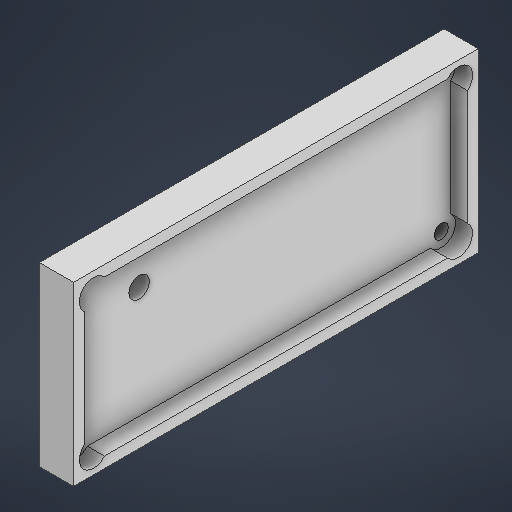
# Autodesk Inventor part: wb_box2026_lid1
Saved by Autodesk Inventor 2027.1 (Build 311270010, 270A)
## iProperties
Created: 2022-08-26
Part Number: wb_box2026_lid1
Material: Générique
Document SubType Name: Modeling
Designer: PCA
Density: 1 g/cm^3
Appearance: Par défaut
Author: PCA
Autodesk Inventor part; units mm, degrees
ref_plane "YZ Plane" through (0, 0, 0) normal (1, 0, 0) x (0, 1, 0)
ref_plane "XZ Plane" through (0, 0, 0) normal (0, 1, 0) x (-1, 0, 0)
ref_plane "XY Plane" through (0, 0, 0) normal (0, 0, 1) x (1, 0, 0)
sketch "Esquisse1" plane through (0, 0, 0) normal (1, 0, 0) x (0, 1, 0)
  line L0 (-15.5, -35.5) -> (15.5, -35.5)
  line L1 (15.5, -35.5) -> (15.5, 35.5)
  line L2 (15.5, 35.5) -> (-15.5, 35.5)
  line L3 (-15.5, 35.5) -> (-15.5, -35.5)
  line L4 (-15.5, -35.5) -> (15.5, 35.5) construction
  line L5 (15.5, -35.5) -> (-15.5, 35.5) construction
  point P0 (0, 0)
  dimension "d0" = 31
  dimension "d1" = 71
  constraints: 12 end point, 2 midpoint, 2 parallel, 1 horizontal, 1 perpendicular
  measures "d0" distance of L2.end L1.end
  measures "d1" distance of L1.end L0.end
extrude "Extrusion1" add sketch "Esquisse1" against normal blind 6
sketch "Esquisse2" plane through (0, 0, 0) normal (1, 0, 0) x (0, 0, -1)
  line L0 (33.6, -13.6) -> (-33.6, -13.6)
  line L1 (-33.6, -13.6) -> (-33.6, 13.6)
  line L2 (-33.6, 13.6) -> (33.6, 13.6)
  line L3 (33.6, 13.6) -> (33.6, -13.6)
  line L4 (33.6, -13.6) -> (-33.6, 13.6) construction
  line L5 (-33.6, -13.6) -> (33.6, 13.6) construction
  point P0 (0, 0)
  dimension "d4" = 67.2
  dimension "d5" = 27.2
  constraints: 12 end point, 2 midpoint, 2 parallel, 1 horizontal, 1 perpendicular
  measures "d4" distance of L1.end L2.end
  measures "d5" distance of L0.end L1.end
extrude "Extrusion2" cut sketch "Esquisse2" against normal blind 3
sketch "Esquisse3" plane through (0, 0, 0) normal (1, 0, 0) x (0, 0, -1)
  line L0 (32, -12) -> (-32, 12) construction
  line L1 (-32, -12) -> (32, 12) construction
  arc A0 (-30.0791, 13.6) -> (-33.6, 10.0791) centre (-32, 12) ccw
  arc A1 (33.5, 10) -> (30, 13.5) centre (32, 12) ccw
  arc A2 (30.0791, -13.6) -> (33.6, -10.0791) centre (32, -12) ccw
  line L2 (-33.6, 13.6) -> (33.6, 13.6) projected
  line L3 (33.6, -13.6) -> (-33.6, 13.6) construction
  line L4 (-33.5, -13.5) -> (33.5, 13.5) construction
  arc A3 (-33.5, -10) -> (-30, -13.5) centre (-32, -12) ccw
  line L5 (-33.6, 13.6) -> (-30.0791, 13.6)
  line L6 (30, 13.5) -> (33.5, 13.5)
  line L7 (-33.5, -13.5) -> (-33.5, -10)
  line L8 (-33.6, 10.0791) -> (-33.6, 13.6)
  line L9 (33.6, -13.6) -> (30.0791, -13.6)
  line L10 (-30, -13.5) -> (-33.5, -13.5)
  line L11 (33.5, 13.5) -> (33.5, 10)
  line L12 (33.6, -10.0791) -> (33.6, -13.6)
  point P0 (0, 0)
  point P1 (33.5, 13.5)
  point P2 (30.0791, 13.6)
  point P3 (-30.0791, 13.6)
  dimension "d8" = 64
  dimension "d9" = 24
  dimension "d10" = 5
  dimension "d12" = 5
  dimension "d13" = 5
  constraints: 24 end point, 8 parallel, 8 point on circle, 4 centre point, 4 coincident, 4 midpoint, 4 perpendicular, 2 horizontal
  measures "d8" distance of L0.end L1.end
  measures "d9" distance of L1.start L0.end
  measures "d10" diameter of A0
  measures "d12" diameter of A1
  measures "d13" diameter of A2
extrude "Extrusion3" cut sketch "Esquisse3" against normal blind 3
sketch "Esquisse4" plane through (-6, 0, 0) normal (-1, 0, 0) x (0, 0, 1)
  line L0 (-28.9525, 9.2685) -> (3.8656, 9.2685) construction
  line L1 (3.8656, 9.2685) -> (3.8656, -1.9036) construction
  line L2 (3.8656, -1.9036) -> (-28.9525, -1.9036) construction
  line L3 (-28.9525, -1.9036) -> (-28.9525, 9.2685) construction
  line L4 (8.1238, -3.2547) -> (23.4156, -3.2547) construction
  line L5 (23.4156, -3.2547) -> (23.4156, -10.1675) construction
  line L6 (23.4156, -10.1675) -> (8.1238, -10.1675) construction
  line L7 (8.1238, -10.1675) -> (8.1238, -3.2547) construction
  line L8 (-28.297, 3.0616) -> (-28.297, 9.1616)
  line L9 (-28.297, 9.1616) -> (-25.9955, 9.1616)
  spline S0 degree 2 poles (-25.9955, 9.1616) (-25.3865, 9.1616) (-25.0657, 9.1012) knots 0 0 0 1 1 1
  spline S1 degree 2 poles (-25.0657, 9.1012) (-24.6147, 9.0268) (-24.0102, 8.6083) (-23.6383, 7.8505) (-23.6383, 7.3948) knots 0 0 0 1 2 3 3 3
  spline S2 degree 2 poles (-23.6383, 7.3948) (-23.6383, 6.6184) (-24.6286, 5.5397) (-25.9211, 5.5397) knots 0 0 0 1 2 2 2
  line L10 (-25.9211, 5.5397) -> (-27.488, 5.5397)
  line L11 (-27.488, 5.5397) -> (-27.488, 3.0616)
  line L12 (-27.488, 3.0616) -> (-28.297, 3.0616)
  line L13 (-27.488, 6.2604) -> (-25.9118, 6.2604)
  spline S3 degree 2 poles (-25.9118, 6.2604) (-25.1261, 6.2604) (-24.4705, 6.8416) (-24.4705, 7.3716) knots 0 0 0 1 2 2 2
  spline S4 degree 2 poles (-24.4705, 7.3716) (-24.4705, 7.7528) (-24.8564, 8.3015) (-25.1726, 8.3852) knots 0 0 0 1 2 2 2
  spline S5 degree 2 poles (-25.1726, 8.3852) (-25.3772, 8.441) (-25.9258, 8.441) knots 0 0 0 1 1 1
  line L14 (-25.9258, 8.441) -> (-27.488, 8.441)
  line L15 (-27.488, 8.441) -> (-27.488, 6.2604)
  line L16 (-18.2589, 5.205) -> (-17.45, 5.0004)
  spline S6 degree 2 poles (-17.45, 5.0004) (-17.7057, 4.0054) (-19.0214, 2.9593) (-19.9746, 2.9593) knots 0 0 0 1 2 2 2
  spline S7 degree 2 poles (-19.9746, 2.9593) (-20.9602, 2.9593) (-22.197, 3.7637) (-22.8432, 5.284) (-22.8432, 6.1581) knots 0 0 0 1 2 3 3 3
  spline S8 degree 2 poles (-22.8432, 6.1581) (-22.8432, 7.1112) (-22.1133, 8.5339) (-20.7696, 9.2685) (-19.9606, 9.2685) knots 0 0 0 1 2 3 3 3
  spline S9 degree 2 poles (-19.9606, 9.2685) (-19.0447, 9.2685) (-17.7987, 8.334) (-17.5522, 7.4925) knots 0 0 0 1 2 2 2
  line L17 (-17.5522, 7.4925) -> (-18.3473, 7.3019)
  spline S10 degree 2 poles (-18.3473, 7.3019) (-18.5612, 7.9667) (-19.3655, 8.5758) (-19.9792, 8.5758) knots 0 0 0 1 2 2 2
  spline S11 degree 2 poles (-19.9792, 8.5758) (-20.6813, 8.5758) (-21.6298, 7.9016) (-22.011, 6.7672) (-22.011, 6.1628) knots 0 0 0 1 2 3 3 3
  spline S12 degree 2 poles (-22.011, 6.1628) (-22.011, 5.3863) (-21.5554, 4.224) (-20.6022, 3.6521) (-20.0443, 3.6521) knots 0 0 0 1 2 3 3 3
  spline S13 degree 2 poles (-20.0443, 3.6521) (-19.3655, 3.6521) (-18.4263, 4.4332) (-18.2589, 5.205) knots 0 0 0 1 2 2 2
  line L18 (-17.1198, 3.0616) -> (-14.7766, 9.1616)
  line L19 (-14.7766, 9.1616) -> (-13.9025, 9.1616)
  line L20 (-13.9025, 9.1616) -> (-11.4104, 3.0616)
  line L21 (-11.4104, 3.0616) -> (-12.331, 3.0616)
  line L22 (-12.331, 3.0616) -> (-13.0377, 4.9074)
  line L23 (-13.0377, 4.9074) -> (-15.5948, 4.9074)
  line L24 (-15.5948, 4.9074) -> (-16.2644, 3.0616)
  line L25 (-16.2644, 3.0616) -> (-17.1198, 3.0616)
  line L26 (-15.3624, 5.563) -> (-13.2888, 5.563)
  line L27 (-13.2888, 5.563) -> (-13.9304, 7.2554)
  spline S14 degree 2 poles (-13.9304, 7.2554) (-14.2186, 8.0272) (-14.3581, 8.52) knots 0 0 0 1 1 1
  spline S15 degree 2 poles (-14.3581, 8.52) (-14.479, 7.9342) (-14.6882, 7.353) knots 0 0 0 1 1 1
  line L28 (-14.6882, 7.353) -> (-15.3624, 5.563)
  line L29 (8.0842, -9.3547) -> (10.1406, -3.2547)
  line L30 (10.1406, -3.2547) -> (11.1392, -3.2547)
  line L31 (11.1392, -3.2547) -> (13.1956, -9.3547)
  line L32 (13.1956, -9.3547) -> (12.3404, -9.3547)
  line L33 (12.3404, -9.3547) -> (11.7867, -7.6493)
  line L34 (11.7867, -7.6493) -> (9.4585, -7.6493)
  line L35 (9.4585, -7.6493) -> (8.9048, -9.3547)
  line L36 (8.9048, -9.3547) -> (8.0842, -9.3547)
  line L37 (11.5643, -6.9573) -> (10.6201, -4.0852)
  line L38 (10.6201, -4.0852) -> (9.6809, -6.9573)
  line L39 (9.6809, -6.9573) -> (11.5643, -6.9573)
  line L40 (18.2229, -9.3547) -> (17.17, -9.3547)
  line L41 (17.17, -9.3547) -> (14.9406, -6.5173)
  line L42 (14.9406, -6.5173) -> (14.5846, -6.9177)
  line L43 (14.5846, -6.9177) -> (14.5846, -9.3547)
  line L44 (14.5846, -9.3547) -> (13.7739, -9.3547)
  line L45 (13.7739, -9.3547) -> (13.7739, -3.2547)
  line L46 (13.7739, -3.2547) -> (14.5846, -3.2547)
  line L47 (14.5846, -3.2547) -> (14.5846, -6.0576)
  line L48 (14.5846, -6.0576) -> (17.0859, -3.2547)
  line L49 (17.0859, -3.2547) -> (18.0746, -3.2547)
  line L50 (18.0746, -3.2547) -> (15.5486, -5.9785)
  line L51 (15.5486, -5.9785) -> (18.2229, -9.3547)
  line L52 (18.0499, -9.3547) -> (20.1063, -3.2547)
  line L53 (20.1063, -3.2547) -> (21.1048, -3.2547)
  line L54 (21.1048, -3.2547) -> (23.1612, -9.3547)
  line L55 (23.1612, -9.3547) -> (22.306, -9.3547)
  line L56 (22.306, -9.3547) -> (21.7524, -7.6493)
  line L57 (21.7524, -7.6493) -> (19.4241, -7.6493)
  line L58 (19.4241, -7.6493) -> (18.8705, -9.3547)
  line L59 (18.8705, -9.3547) -> (18.0499, -9.3547)
  line L60 (21.5299, -6.9573) -> (20.5858, -4.0852)
  line L61 (20.5858, -4.0852) -> (19.6466, -6.9573)
  line L62 (19.6466, -6.9573) -> (21.5299, -6.9573)
  point P0 (0, 0)
  constraints: 4 other
extrude "Extrusion4" add sketch "Esquisse4" along normal blind 1
sketch "Esquisse5" plane through (-6, 0, 0) normal (-1, 0, 0) x (0, 0, 1)
  arc A0 (-30.0791, 13.6) -> (-33.6, 10.0791) centre (-32, 12) ccw projected
  line L0 (32, -12) -> (-32, -12)
  line L1 (-32, -12) -> (-32, 12)
  line L2 (-32, 12) -> (32, 12)
  line L3 (32, 12) -> (32, -12)
  line L4 (32, -12) -> (-32, 12) construction
  line L5 (-32, -12) -> (32, 12) construction
  circle A1 centre (-32, 12) radius 1.25
  circle A2 centre (-32, -12) radius 1.25
  circle A3 centre (32, 12) radius 1.25
  circle A4 centre (32, -12) radius 1.25
  line L6 (35.5, 15.5) -> (-35.5, 15.5) projected
  line L7 (35.5, -15.5) -> (35.5, 15.5) projected
  point P0 (0, 0)
  dimension "d18" = 64
  dimension "d19" = 24
  dimension "d20" = 2.5
  dimension "d21" = 2.5
  dimension "d22" = 2.5
  dimension "d24" = 2.5
  constraints: 12 end point, 4 centre point, 3 coincident, 2 midpoint, 2 parallel, 1 horizontal, 1 perpendicular, 1 point on line
  measures "d18" distance of L1.end L2.end
  measures "d19" distance of L0.end L1.end
  measures "d20" diameter of A1
  measures "d21" diameter of A2
  measures "d22" diameter of A3
  measures "d24" diameter of A4
hole "Perçage1" at (-6, 12, 32) at (-6, -12, -32) at (-6, -12, 32) at (-6, 12, -32) direction (1, 0, 0) diameter 2.5 end through all
sketch "Esquisse6" plane through (-6, 0, 0) normal (-1, 0, 0) x (0, 0, 1)
  circle A0 centre (21, 6) radius 1.8
  line L0 (35.5, 15.5) -> (-35.5, 15.5) projected
  line L1 (35.5, -15.5) -> (35.5, 15.5) projected
  point P0 (0, 0)
  dimension "d37" = 3.6
  dimension "d38" = 9.5
  dimension "d39" = 14.5
  constraints: 1 centre point
  measures "d37" diameter of A0
  measures "d38" distance from line of L0 A0.centre
  measures "d39" distance from line of L1 A0.centre
extrude "Extrusion5" cut sketch "Esquisse6" against normal blind 10
